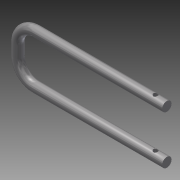
# Autodesk Inventor part: GARFO
Saved by Autodesk Inventor 2015 (Build 190159000, 159)
## iProperties
Created: 2016-08-09
Part Number: GARFO
Material: Aluminium AW-7020
Document SubType Name: Modeling
Designer: EriveltonDell
Density: 2.78 g/cm^3
Appearance: Stainless - Brushed
Mass: 1234.07 g
Surface Area: 731.335 cm^2
Volume: 443.911 cm^3
Author: EriveltonDell
Autodesk Inventor part; units mm, degrees
ref_plane "YZ Plane" through (0, 0, 0) normal (1, 0, 0) x (0, 1, 0)
ref_plane "XZ Plane" through (0, 0, 0) normal (0, 1, 0) x (-1, 0, 0)
ref_plane "XY Plane" through (0, 0, 0) normal (0, 0, 1) x (1, 0, 0)
sketch "Sketch1" plane through (0, 0, 0) normal (0, 1, 0) x (-1, 0, 0)
  line L0 (0, 0) -> (350, 0)
  line L1 (400, 50) -> (400, 80)
  line L2 (350, 130) -> (0, 130)
  arc A0 (350, 0) -> (400, 50) centre (350, 50) ccw
  arc A1 (400, 80) -> (350, 130) centre (350, 80) ccw
  point P0 (400, 0)
  point P1 (400, 130)
  dimension "d7" = 400
  dimension "d8" = 130
  dimension "d9" = 400
  dimension "d10" = 50
  constraints: 6 end point, 4 point on circle, 4 point on line, 4 tangent, 2 centre point, 2 perpendicular, 1 equal radius, 1 horizontal
  measures "d7" distance of L0.start point (400, 0)
  measures "d8" distance of point (400, 0) point (400, 130)
  measures "d9" distance of point (400, 130) L2.end
  measures "d10" radius of A0
sketch "Sketch2" plane through (0, 0, 0) normal (1, 0, 0) x (0, 1, 0)
  circle A0 centre (0, 0) radius 12.7
  dimension "d11" = 25.4
  constraints: 1 centre point, 1 coincident
  measures "d11" diameter of A0
sweep "Sweep1" add profiles "Sketch2" path "Sketch1" path curves L0 A0 L1 A1 L2
sketch "Sketch3" plane through (0, 0, 0) normal (0, 0, 1) x (1, 0, 0)
  line L0 (0, 0) -> (-30, 0)
  circle A0 centre (-30, 0) radius 6
  dimension "d14" = 30
  dimension "d15" = 12
  constraints: 2 end point, 1 centre point, 1 coincident, 1 horizontal
  measures "d14" distance of L0.start L0.end
  measures "d15" diameter of A0
extrude "Extrusion1" cut sketch "Sketch3" along normal through all both and the other way through all
body "Solid1"
